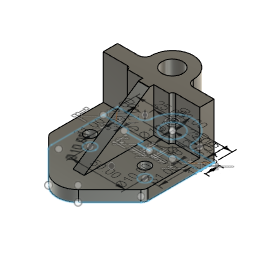
Lab 3 A3 (Autodesk Fusion 360 design; units mm, degrees)
Autodesk Fusion 360 part; units mm, degrees
sketch "Sketch1" plane through (0, 0, 0) normal (0, 0, 1) x (1, 0, 0)
  line L0 (-44, -10.6757) -> (-44, 49.5)
  line L1 (44, 49.5) -> (44, -10.6757)
  circle A0 centre (0, 55.5) radius 9.5
  line L2 (44, 49.5) -> (44, 36.5)
  line L3 (-44, 49.5) -> (-25, 49.5)
  line L4 (25, 49.5) -> (44, 49.5)
  arc A1 (-25, 49.5) -> (-19, 55.5) centre (-25, 55.5) ccw
  arc A2 (19, 55.5) -> (25, 49.5) centre (25, 55.5) ccw
  arc A3 (19, 55.5) -> (-19, 55.5) centre (0, 55.5) ccw
  line L5 (44, 36.5) -> (22, 36.5)
  line L6 (-22, 36.5) -> (-44, 36.5)
  arc A4 (22, 36.5) -> (19, 33.502) centre (22, 33.5) ccw
  arc A5 (-19, 33.502) -> (-22, 36.5) centre (-22, 33.5) ccw
  line L7 (5, 33.502) -> (5, 29.502)
  line L8 (5, 29.502) -> (-5, 29.502)
  line L9 (-5, 29.502) -> (-5, 33.502)
  line L10 (19, 33.502) -> (5, 33.502)
  line L11 (-5, 33.502) -> (-19, 33.502)
  circle A6 centre (-25, 5.5) radius 5
  circle A7 centre (25, 5.5) radius 5
  line L12 (-5, 29.502) -> (5, 29.502)
  line L13 (-13.435, -43.933) -> (-42.0962, -15.2719)
  line L14 (13.435, -43.933) -> (42.0962, -15.2719)
  arc A8 (-44, -10.6757) -> (-42.0962, -15.2719) centre (-37.5, -10.6757) ccw
  arc A9 (42.0962, -15.2719) -> (44, -10.6757) centre (37.5, -10.6757) ccw
  arc A10 (-13.63, -43.7381) -> (13.63, -43.7381) centre (0, -30.498) ccw
  line L15 (32.4444, 36.5) -> (44, 49.5) construction
  line L16 (-32.4444, 36.5) -> (-44, 49.5) construction
  dimension "d1" = 88
  dimension "d3" = 12
  dimension "d4" = 6
  dimension "d5" = 12
  dimension "d6" = 6
  dimension "d7" = 19
  dimension "d8" = 38
  dimension "d9" = 25
  dimension "d10" = 25
  dimension "d11" = 13
  dimension "d15" = 6
  dimension "d16" = 6
  dimension "d17" = 3
  dimension "d19" = 3
  dimension "d21" = 10
  dimension "d22" = 4
  dimension "d23" = 39
  dimension "d24" = 10
  dimension "d25" = 10
  dimension "d26" = 50
  dimension "d27" = 31
  dimension "d28" = 31
  dimension "d29" = 19
  dimension "d37" = 10
  dimension "d39" = 19
  dimension "d41" = 19
  dimension "d42" = 13
  dimension "d43" = 13
  dimension "d44" = 6.5
  dimension "d45" = 6.5
  dimension "d46" = 6.5
  dimension "d47" = 6.5
  constraint parallel L0 L1
  constraint concentric A0 A3
  constraint perpendicular L2 L3
  constraint coincident L0 L6.end
  constraint perpendicular L0 L5
  constraint horizontal L10
  constraint collinear L3 L4
  constraint collinear L5 L6
  constraint vertical L7
  constraint horizontal L8
  constraint vertical L9
  constraint coincident L9.end L10
  constraint collinear L10 L11
  constraint horizontal L12
  constraint coincident L14 A10.end
  constraint coincident L13 A10.start
  constraint coincident L5 L15.start
  constraint coincident L6 L16.start
  measures "d1" distance of L0.end L1.start
  measures "d3" diameter of A2
  measures "d4" distance of A2.centre L3
  measures "d5" diameter of A1
  measures "d6" distance of A1.centre L3
  measures "d7" diameter of A0
  measures "d8" diameter of A3
  measures "d9" distance of A2.centre A0.centre
  measures "d10" distance of A1.centre A0.centre
  measures "d11" distance of L1.start L2.end
  measures "d15" diameter of A5
  measures "d16" diameter of A4
  measures "d17" distance of A5.centre L5
  measures "d19" distance of A4.centre L5
  measures "d21" distance of L9.end L7.start
  measures "d22" distance of L9.end L8.end
  measures "d23" distance of L0 L9
  measures "d24" diameter of A6
  measures "d25" diameter of A7
  measures "d26" horizontal distance of A6.centre A7.centre
  measures "d27" distance of L5 A7.centre
  measures "d28" distance of L6 A6.centre
  measures "d29" distance of L0 A6.centre
  measures "d37" distance of L8.end L7.end
  measures "d39" distance of A10.centre L14.start
  measures "d41" distance of A10.centre L13.start
  measures "d42" diameter of A9
  measures "d43" diameter of A8
  measures "d44" distance of L0 A8.centre
  measures "d45" distance of L13 A8.centre
  measures "d46" distance of L1 A9.centre
  measures "d47" distance of L14 A9.centre
extrude "Extrude1" add sketch "Sketch1" along normal blind 10 contours L0 L1 L5 L6 A4 A5 L7 L8 L9 L10 L11 L12 L13 L14 A8 A9 A10
extrude "Extrude2" add sketch "Sketch1" along normal blind 50 contours L0 L1 L2 L3 L4 A1 A2 A3 L5 L6 A4 A5 L7 L8 L9 L10 L11 L12
sketch "Sketch2" plane through (0, 0, 0) normal (1, 0, 0) x (0, 1, 0)
  line L0 (30, 50) -> (30, 10)
  line L1 (30, 10) -> (-30, 10)
  line L2 (-30, 10) -> (30, 50)
  dimension "d52" = 60
  constraint vertical L0
  constraint perpendicular L0 L1
  measures "d52" distance of L0.end L1.end
extrude "Extrude3" add sketch "Sketch2" along normal mid plane 10
extrude "Extrude4" add sketch "Sketch1" along normal blind 10 contours L0 L1 L2 L3 L4 A1 A2 A3 L5 L6 A4 A5 L7 L8 L9 L10 L11 L12 | A0
delete_face "DeleteFace1" 1 faces at (2.462, 58.5873, 10)
